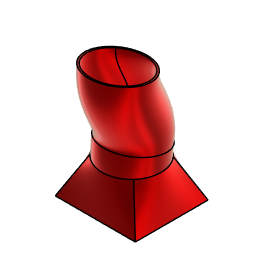
Tolva+de+alimentacion (Autodesk Fusion 360 design; units mm, degrees)
Autodesk Fusion 360 part; units mm, degrees
sketch "Boceto1" plane through (0, 0, 0) normal (0, 0, 1) x (1, 0, 0)
  circle A0 centre (0, 0) radius 30
  circle A1 centre (0, 0) radius 32
  dimension "d12" = 2
  dimension "d13" = 60
  constraint coincident A0.centre A1.centre
  measures "d12" distance of A0 A1
  measures "d13" diameter of A0
ref_plane "PlanoDeObra1" through (0, 0, -40) normal (0, 0, 1) x (1, 0, 0)
sketch "Boceto2" plane through (0, 0, -40) normal (0, 0, 1) x (1, 0, 0)
  line L0 (-40, 36) -> (-40, -36)
  line L1 (40, 36) -> (40, -36)
  line L2 (-40, 36) -> (40, 36)
  line L3 (-40, -36) -> (40, -36)
  line L4 (43.5, 39.5) -> (43.5, -39.5)
  line L5 (-43.5, -39.5) -> (43.5, -39.5)
  line L6 (-43.5, 39.5) -> (-43.5, -39.5)
  line L7 (-43.5, 39.5) -> (43.5, 39.5)
  line L8 (0, 36) -> (0, -36) construction
  dimension "d2" = 3.5
  dimension "d4" = 72
  dimension "d5" = 87
  constraint vertical L1
  constraint horizontal L2
  constraint horizontal L3
  constraint vertical L0
  constraint midpoint L2 L8.start
  constraint midpoint L3 L8.end
  constraint midpoint L8 origin
  measures "d4" distance of L1.start L1.end
  measures "d5" distance of L4.start L6.start
loft "Solevación1" add profiles "Boceto2", "Boceto1" section 1 section 2
loft "Solevación2" cut profiles "Boceto2", "Boceto1" section 1 contours L0 L1 L2 L3 section 2 contours A0
sketch "Boceto5" plane through (0, 0, 0) normal (1, 0, 0) x (0, 1, 0)
  arc A0 (1.4235, 16.2702) -> (0, 0) centre (93.6965, 0) ccw
  dimension "d22" = 10
  constraint coincident A0.end origin
  constraint horizontal A0.end A0.centre
  measures "d22" angle of A0.end A0.start A0.centre
sweep "Barrido1" add 1 faces at (24.1943, 19.793, 0) path "Boceto5" along A0
sketch "Boceto6" plane through (0, 0, 0) normal (1, 0, 0) x (0, 1, 0)
  arc A0 (1.4235, 16.2702) -> (0, 0) centre (93.6965, 0) ccw
  line L0 (-14.758, 90.6645) -> (-25.6524, 20.4726) construction
  line L1 (-25.6524, 20.4726) -> (1.4235, 16.2702) construction
  spline S0 degree 5 poles (-14.758, 90.6645) (-15.0151, 89.0086) (-15.3594, 85.682) (-15.3667, 80.6478) (-14.4239, 73.8789) (-12.0247, 65.4963) (-8.8804, 57.4) (-5.4982, 49.7683) (-2.3587, 42.6952) (0.1604, 36.091) (1.7957, 29.6992) (2.2467, 24.5147) (2.049, 20.4682) (1.6727, 17.684) (1.4235, 16.2702) knots 0 0 0 0 0 0 0.1 0.2 0.3 0.4 0.5 0.6 0.7 0.8 0.9 1 1 1 1 1 1
  line L2 (3.1484, 26.0527) -> (-0.3015, 6.4877)
  point P0 (1.4235, 16.2702)
  point P1 (-4.056, 46.4663)
  dimension "d23" = 27.4
  constraint coincident P0 A0.start
  constraint perpendicular L0 L1
  constraint midpoint P0 L2
  constraint tangent A0 L2
  measures "d23" distance of L0.end P0
sweep "Barrido2" add 1 faces at (4.2954, -29.0665, 21.6464) path "Boceto6" along S0
sketch "Boceto4" plane through (0, 0, 0) normal (1, 0, 0) x (0, 1, 0)
  circle A0 centre (0, -70) radius 20.5
  line L0 (23, -70) -> (-23, -70)
  dimension "d3" = 41
  constraint vertical A0.centre origin
  constraint coincident A0.centre L0
  measures "d3" diameter of A0
extrude "Extruir1" [suppressed]
equation "d4 = 79 mm - 2 * d2"
equation "d5 = 80 mm + 2 * d2"
